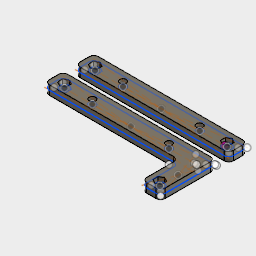
Anet_A8_power_supply_adapter_for_Meanwell_LRS-350 (Autodesk Fusion 360 design; units mm, degrees)
Autodesk Fusion 360 part; units mm, degrees
sketch "Sketch1" plane through (0, 0, 0) normal (0, 1, 0) x (1, 0, 0)
  circle A0 centre (1.6, 0) radius 1.6
  line L0 (0, 0) -> (-83, 0) construction
  circle A1 centre (-84.6, 0) radius 1.6
  line L1 (-81.8, 1.6166) -> (-84.6, 3.2332)
  line L2 (-84.6, 3.2332) -> (-87.4, 1.6166)
  line L3 (-87.4, 1.6166) -> (-87.4, -1.6166)
  line L4 (-87.4, -1.6166) -> (-84.6, -3.2332)
  line L5 (-84.6, -3.2332) -> (-81.8, -1.6166)
  line L6 (-81.8, -1.6166) -> (-81.8, 1.6166)
  line L7 (4.4, 1.6166) -> (1.6, 3.2332)
  line L8 (1.6, 3.2332) -> (-1.2, 1.6166)
  line L9 (-1.2, 1.6166) -> (-1.2, -1.6166)
  line L10 (-1.2, -1.6166) -> (1.6, -3.2332)
  line L11 (1.6, -3.2332) -> (4.4, -1.6166)
  line L12 (4.4, -1.6166) -> (4.4, 1.6166)
  circle A2 centre (-16.4, 0) radius 2.1
  circle A3 centre (-66.4, 0) radius 2.1
  line L13 (-66.4, 0) -> (-16.4, 0) construction
  line L14 (5.6, 6) -> (-88.4, 6)
  line L15 (-91.4, 3) -> (-91.4, -3)
  line L16 (-88.4, -6) -> (5.6, -6)
  line L17 (8.6, -3) -> (8.6, 3)
  line L18 (8.6, 6) -> (-91.4, -6) construction
  line L19 (-91.4, 6) -> (8.6, -6) construction
  arc A4 (-88.4, 6) -> (-91.4, 3) centre (-88.4, 3) ccw
  arc A5 (-91.4, -3) -> (-88.4, -6) centre (-88.4, -3) ccw
  arc A6 (8.6, 3) -> (5.6, 6) centre (5.6, 3) ccw
  arc A7 (5.6, -6) -> (8.6, -3) centre (5.6, -3) ccw
  dimension "d1" = 3.2
  dimension "d2" = 83
  dimension "d3" = 3.2
  dimension "d4" = 4.2
  dimension "d5" = 18
  dimension "d6" = 4.2
  dimension "d7" = 50
  dimension "d8" = 100
  dimension "d9" = 12
  dimension "d22" = 3
  constraint coincident L0.start A0
  constraint coincident L0.start origin
  constraint coincident L0.start A1
  constraint coincident L0 origin
  constraint perpendicular L14 L15
  constraint parallel L14 L16
  constraint parallel L15 L17
  constraint horizontal L14
  constraint coincident L18 L0.start
  constraint coincident L19 L0.start
  constraint midpoint L13 L0.start
  constraint coincident L0.start L14
  constraint coincident L0.start L15
  constraint tangent L14 A4
  constraint tangent L15 A4
  constraint coincident L0.start L16
  constraint tangent L15 A5
  constraint tangent L16 A5
  constraint equal A4 A5
  constraint tangent L14 A6
  constraint tangent L17 A6
  constraint equal A4 A6
  constraint coincident L0.start L17
  constraint tangent L16 A7
  constraint tangent L17 A7
  constraint equal A4 A7
  measures "d1" diameter of A0
  measures "d3" diameter of A1
  measures "d4" diameter of A2
  measures "d6" diameter of A3
  measures "d22" radius of A4
extrude "Extrude5" add sketch "Sketch1" along normal blind 3 and the other way blind 3 contours L14 L15 L16 L17 A4 A5 A6 A7 makes body 1
extrude "Extrude6" add sketch "Sketch1" along normal blind -3 and the other way blind 1 contours L1 L2 L3 L4 L5 L6 | L7 L8 L9 L10 L11 L12 bodies 1
chamfer "Chamfer1" distance 2.5 angle 45 1 edges at (-18.3579, -3, 0.7594) measured on face at (-49.681, -3, 4.698) on bodies 1
chamfer "Chamfer2" distance 2.5 angle 45 1 edges at (-68.3579, -3, 0.7594) measured on face at (-2.2093, -3, 3.5048) on bodies 1
sketch "Sketch2" plane through (0, 0, 0) normal (0, 1, 0) x (1, 0, 0)
  circle A0 centre (-66.4, -20) radius 2.1
  line L0 (-66.4, -20) -> (-16.4, -20) construction
  arc A1 (-91.4, -23) -> (-88.4, -26) centre (-88.4, -23) ccw
  line L1 (8.6, -14) -> (-91.4, -26) construction
  line L2 (0, -20) -> (-83, -20) construction
  line L3 (-84.6, -16.7668) -> (-87.4, -18.3834)
  arc A2 (6.7365, -25.7764) -> (7.6, -25.2361) centre (5.6, -23) ccw
  line L4 (4.6, -14) -> (-88.4, -14)
  line L5 (-87.4, -18.3834) -> (-87.4, -21.6166)
  line L6 (-81.8, -18.3834) -> (-84.6, -16.7668)
  line L7 (-91.4, -14) -> (8.6, -26) construction
  line L8 (-91.4, -17) -> (-91.4, -23)
  line L9 (-81.8, -21.6166) -> (-81.8, -18.3834)
  line L10 (-87.4, -21.6166) -> (-84.6, -23.2332)
  circle A3 centre (-16.4, -20) radius 2.1
  arc A4 (-88.4, -14) -> (-91.4, -17) centre (-88.4, -17) ccw
  circle A5 centre (-84.6, -20) radius 1.6
  line L11 (-84.6, -23.2332) -> (-81.8, -21.6166)
  line L12 (1.6, -20) -> (1.6, -44) construction
  circle A6 centre (1.6, -44) radius 1.6
  line L13 (4.4, -42.3834) -> (1.6, -40.7668)
  line L14 (1.6, -40.7668) -> (-1.2, -42.3834)
  line L15 (-1.2, -42.3834) -> (-1.2, -45.6166)
  line L16 (-1.2, -45.6166) -> (1.6, -47.2332)
  line L17 (1.6, -47.2332) -> (4.4, -45.6166)
  line L18 (4.4, -45.6166) -> (4.4, -42.3834)
  line L19 (4.6, -49.5) -> (-1.4, -49.5)
  line L20 (7.6, -17) -> (7.6, -46.5)
  line L21 (7.6, -49.5) -> (-4.4, -14.5) construction
  line L22 (-4.4, -49.5) -> (7.6, -14.5) construction
  line L23 (-88.4, -26) -> (-7.4, -26)
  line L24 (-4.4, -46.5) -> (-4.4, -29)
  line L25 (7.6, -14.5) -> (7.6, -14)
  arc A7 (-4.4, -29) -> (-7.4, -26) centre (-7.4, -29) ccw
  arc A8 (-4.4, -46.5) -> (-1.4, -49.5) centre (-1.4, -46.5) ccw
  arc A9 (4.6, -49.5) -> (7.6, -46.5) centre (4.6, -46.5) ccw
  arc A10 (7.6, -17) -> (4.6, -14) centre (4.6, -17) ccw
  dimension "d37" = 3.2
  dimension "d38" = 4.2
  dimension "d39" = 18
  dimension "d40" = 4.2
  dimension "d41" = 50
  dimension "d42" = 100
  dimension "d43" = 12
  dimension "d44" = 3
  dimension "d45" = 24
  dimension "d46" = 3.2
  dimension "d47" = 12
  dimension "d48" = 35
  dimension "d49" = 3
  dimension "d50" = 3
  dimension "d51" = 3
  constraint coincident origin A5
  constraint coincident origin L2
  constraint perpendicular L4 L8
  constraint parallel L4 L23
  constraint horizontal L4
  constraint coincident origin L1
  constraint coincident origin L7
  constraint midpoint origin L0
  constraint coincident L4
  constraint coincident L8
  constraint tangent L4 A4
  constraint tangent L8 A4
  constraint coincident L23
  constraint tangent A1 L8
  constraint tangent A1 L23
  constraint equal A1 A4
  constraint tangent A2 L23
  constraint perpendicular L19 L24
  constraint parallel L20 L24
  constraint horizontal L19
  constraint coincident L21 origin
  constraint coincident L22 origin
  constraint midpoint L12 origin
  constraint coincident L20
  constraint coincident L7 origin
  constraint tangent L23 A7
  constraint tangent L24 A7
  constraint coincident L19
  constraint coincident L24
  constraint tangent L19 A8
  constraint tangent L24 A8
  constraint tangent L20 A9
  constraint tangent L19 A9
  constraint equal A8 A9
  constraint coincident origin L20
  constraint tangent L4 A10
  constraint tangent L20 A10
  measures "d37" diameter of A5
  measures "d38" diameter of A3
  measures "d40" diameter of A0
  measures "d44" radius of A4
  measures "d46" diameter of A6
  measures "d48" distance of origin
  measures "d49" radius of A7
  measures "d50" radius of A8
  measures "d51" radius of A10
extrude "Extrude7" add sketch "Sketch2" along normal blind 3 and the other way blind 3 separate body contours A1 L4 L8 A4 L19 L20 L23 L24 A7 A8 A9 A10 makes body 2
extrude "Extrude8" add sketch "Sketch2" along normal blind -1 and the other way blind 3 contours L3 L5 L6 L9 L10 L11 | L13 L14 L15 L16 L17 L18 bodies 2
chamfer "Chamfer3" distance 2.5 angle 45 1 edges at (-68.3579, -3, 20.7594) measured on face at (1.8667, -3, 29.5381) on bodies 2
chamfer "Chamfer4" distance 2.5 angle 45 1 edges at (-18.3579, -3, 20.7594) measured on face at (1.8667, -3, 29.5381) on bodies 2
